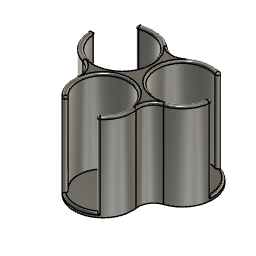
munzhalter-v5 (Autodesk Fusion 360 design; units mm, degrees)
Autodesk Fusion 360 part; units mm, degrees
sketch "Skizze1" plane through (0, 0, 0) normal (0, 0, 1) x (1, 0, 0)
  circle A0 centre (-12.1729, 12.2118) radius 13.25
  circle A1 centre (-12.1729, 12.2118) radius 15.25
  line L0 (-12.1729, 12.2118) -> (16.8271, 12.2118) construction
  circle A2 centre (16.8271, 12.2118) radius 12.5
  circle A3 centre (16.8271, 12.2118) radius 14.5
  line L1 (2.3271, 12.2118) -> (2.8175, 12.2118) construction
  line L2 (2.8175, 12.2118) -> (2.8175, 9.41) construction
  line L3 (2.8175, 9.41) -> (2.3271, 9.41) construction
  line L4 (2.3271, 9.41) -> (2.3271, 12.2118) construction
  line L5 (2.3271, 12.2118) -> (2.8175, 9.41) construction
  line L6 (2.3271, 9.41) -> (2.8175, 12.2118) construction
  line L7 (2.5723, 10.8109) -> (2.5723, 12.2118) construction
  line L8 (2.5723, 12.2118) -> (2.5723, -11.7882) construction
  circle A4 centre (2.5723, -11.7882) radius 12
  circle A5 centre (2.5723, -11.7882) radius 14
  line L9 (2.5723, -11.7882) -> (2.5723, -25.7882) construction
  line L10 (-12.1729, 12.2118) -> (-24.9626, 20.5176) construction
  line L11 (-24.9626, 20.5176) -> (-9.753, 20.5176) construction
  line L12 (-24.9626, 20.5176) -> (-9.753, 20.5176) construction
  line L13 (-12.1729, 12.2118) -> (-28.2192, 22.6324) construction
  line L14 (-28.2192, 22.6324) -> (-24.9626, 20.5176) construction
  line L15 (-24.9626, 20.5176) -> (-20.8778, 26.8076) construction
  line L16 (-20.8778, 26.8076) -> (-29.0474, 14.2275)
  line L17 (-29.0474, 14.2275) -> (-24.4644, 11.2513)
  line L18 (-24.4644, 11.2513) -> (-16.2948, 23.8313)
  line L19 (-16.2948, 23.8313) -> (-20.8778, 26.8076)
  line L20 (2.5723, -25.7882) -> (10.0723, -25.7882) construction
  line L21 (10.0723, -25.7882) -> (-4.9277, -25.7882)
  line L22 (-4.9277, -25.7882) -> (-4.9277, -20.4204)
  line L23 (-4.9277, -20.4204) -> (10.0723, -20.4204)
  line L24 (10.0723, -20.4204) -> (10.0723, -25.7882)
  line L25 (16.8271, 12.2118) -> (28.9878, 20.1091) construction
  line L26 (16.8271, 12.2118) -> (31.3271, 12.2118) construction
  line L27 (28.9878, 20.1091) -> (33.0726, 13.8191) construction
  line L28 (33.0726, 13.8191) -> (24.903, 26.3991)
  line L29 (24.903, 26.3991) -> (20.5571, 23.5769)
  line L30 (20.5571, 23.5769) -> (28.7267, 10.9968)
  line L31 (28.7267, 10.9968) -> (33.0726, 13.8191)
  dimension "d1" = 26.5
  dimension "d2" = 2
  dimension "d5" = 29
  dimension "d6" = 25
  dimension "d7" = 2
  dimension "d8" = 24
  dimension "d9" = 24
  dimension "d10" = 2
  dimension "d22" = 7.5
  dimension "d23" = 15
  dimension "d24" = 7.5
  dimension "d25" = 15
  dimension "d26" = 33
  dimension "d27" = 7.5
  dimension "d28" = 15
  constraint coincident A0.centre A1.centre
  constraint horizontal L0
  constraint coincident L0.end A2.centre
  constraint horizontal L1
  constraint vertical L2
  constraint horizontal L3
  constraint vertical L4
  constraint coincident A1 L2.end
  constraint midpoint L0 L1.start
  constraint midpoint L5 L7.start
  constraint midpoint L1 L7.end
  constraint parallel L7 L8
  constraint coincident L8.end A4.centre
  constraint coincident A5 L9.end
  constraint parallel L8 L9
  constraint coincident A1 L10.end
  constraint horizontal L11
  constraint horizontal L12
  constraint parallel L10 L13
  constraint perpendicular L14 L15
  constraint perpendicular L16 L17
  constraint parallel L16 L18
  constraint parallel L17 L19
  constraint perpendicular L10 L16
  constraint perpendicular L9 L20
  constraint horizontal L21
  constraint vertical L22
  constraint horizontal L23
  constraint vertical L24
  constraint horizontal L26
  constraint perpendicular L25 L27
  constraint perpendicular L28 L29
  constraint parallel L28 L30
  constraint parallel L29 L31
  constraint parallel L27 L28
  measures "d1" diameter of A0
  measures "d5" distance of A0.centre L0.end
  measures "d6" diameter of A2
  measures "d8" distance of L7.end L8.end
  measures "d9" diameter of A4
  measures "d22" distance of L10.end L15.end
  measures "d23" distance of L15.end L16.end
  measures "d24" distance of L9.end L20.end
  measures "d25" distance of L20.end L21.end
  measures "d26" angle of L25 L26
  measures "d27" distance of L25.end L27.end
  measures "d28" distance of L27.end L28.end
extrude "Extrusion1" add sketch "Skizze1" against normal blind 2 contours A0 L17 L18 L19 | A0 A1 A3 A5 L17 L19 | A0 L17 L18 L19 | A0 A1 L17 L19 | A1 A2 A3 A5 L29 L31 | A1 A3 | A1 A5 | A1 A3 A4 A5 L22 L24 | A2 A3 L29 L31 | A1 A3 A5 | A4 A5 L22 L24 | A2 L29 L30 L31 | A2 L29 L30 L31 | A3 A5 | A4 L22 L23 L24 | A4 L22 L23 L24
extrude "Extrusion2" add sketch "Skizze1" along normal blind 40 contours A0 A1 A3 A5 L17 L19 | A1 A2 A3 A5 L29 L31 | A1 A3 | A1 A5 | A1 A3 A4 A5 L22 L24 | A1 A3 A5 | A3 A5
fillet "Abrundung1" radius 7.5 3 edges at (12.0404, -1.4753, 19) (2.7118, 15.5297, 19) (-7.8156, -2.4024, 19)
fillet "Abrundung2" radius 1 12 edges at (10.0723, -23.6098, 20) (10.0723, -21.1557, 20) (-4.9277, -23.6098, 20) (-4.9277, -21.1557, 20) (31.3195, 12.6806, 20) (29.2986, 11.3682, 20) (23.1499, 25.2606, 20) (-19.2242, 25.7337, 20) (-27.3938, 13.1537, 20) (-25.4185, 11.8709, 20) (21.129, 23.9482, 20) (-17.2489, 24.451, 20)
fillet "Abrundung3" radius 1 3 edges at (-24.9626, 20.5176, 0) (2.5723, -25.7882, 0) (28.9878, 20.1091, 0)
fillet "Abrundung4" radius 1 36 edges at (14.15, 26.4625, 40) (21.9449, 24.7441, 40) (6.3437, 5.4038, 40) (30.3575, 11.7898, 40) (28.1407, 3.1426, 40) (17.4455, -4.7221, 40) (15.6964, -16.6623, 40) (10.3157, -22.2782, 40) (2.5723, 0.2118, 40) (-5.1711, -22.2782, 40) (-10.4451, -16.9405, 40) (-12.5586, -5.4057, 40) (-24.1362, 2.7545, 40) (-26.4576, 12.3103, 40) (-1.0605, 4.9954, 40) (-18.073, 25.2215, 40) (-9.3765, 27.2032, 40) (2.758, 21.7484, 40) (6.3437, 5.4038, 40) (30.3575, 11.7898, 40) (28.1407, 3.1426, 40) (17.4455, -4.7221, 40) (15.6964, -16.6623, 40) (10.3157, -22.2782, 40) (2.5723, 0.2118, 40) (-5.1711, -22.2782, 40) (-10.4451, -16.9405, 40) (-12.5586, -5.4057, 40) (-24.1362, 2.7545, 40) (-26.4576, 12.3103, 40) (-1.0605, 4.9954, 40) (-18.073, 25.2215, 40) (-9.3765, 27.2032, 40) (2.758, 21.7484, 40) (14.15, 26.4625, 40) (21.9449, 24.7441, 40)
